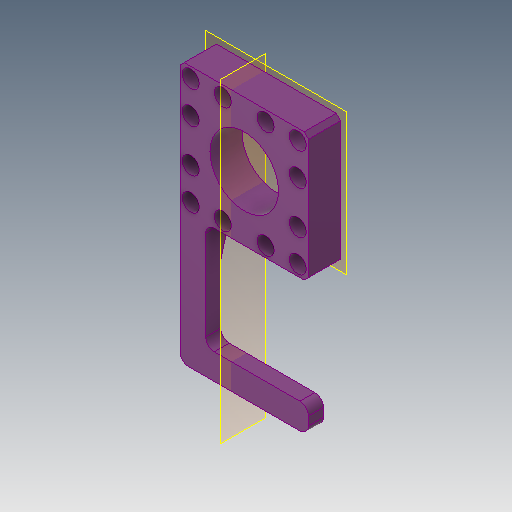
# Autodesk Inventor part: cellSTORM_UC2_Sample_arm
Saved by Autodesk Inventor 2019.4 (Build 234330000, 330)
## iProperties
Created: 2020-12-29
Part Number: cellSTORM_UC2_Sample_arm
Material: Generic
Document SubType Name: Modeling
Designer: diederichbenedict
Density: 1 g/cm^3
Appearance: Smooth - Purple
Author: diederichbenedict
Autodesk Inventor part; units mm, degrees
ref_plane "YZ Plane" through (0, 0, 0) normal (1, 0, 0) x (0, 1, 0)
ref_plane "XZ Plane" through (0, 0, 0) normal (0, 1, 0) x (-1, 0, 0)
ref_plane "XY Plane" through (0, 0, 0) normal (0, 0, 1) x (1, 0, 0)
ref_plane "Work Plane1" through (0, 0, 0) normal (0, 0, 1) x (1, 0, 0)
sketch "Sketch1" plane through (0, 0, 0) normal (0, 0, 1) x (1, 0, 0)
  circle A0 centre (-10, -25) radius 1.45 projected
  circle A1 centre (-10, 25) radius 1.45 projected
  circle A2 centre (10, 25) radius 1.45 projected
  circle A3 centre (10, -25) radius 1.45 projected
  circle A4 centre (-25, 25) radius 2.325 projected
  circle A5 centre (25, -25) radius 2.325 projected
  circle A6 centre (-25, -25) radius 2.325 projected
  circle A7 centre (25, 25) radius 2.325 projected
  line L0 (28, 30) -> (30, 28) projected
  line L1 (28, 30) -> (-28, 30) projected
  line L2 (-30, 28) -> (-28, 30) projected
  line L3 (-30, 28) -> (-30, -28) projected
  line L4 (-28, -30) -> (-30, -28) projected
  line L5 (-28, -30) -> (28, -30) projected
  line L6 (30, -28) -> (28, -30) projected
  line L7 (30, -28) -> (30, 28) projected
  circle A8 centre (-17.5, -17.5) radius 1.95 projected
  circle A9 centre (17.5, 17.5) radius 1.95 projected
  circle A10 centre (17.5, -17.5) radius 1.95 projected
  circle A11 centre (-17.5, 17.5) radius 1.95 projected
  circle A12 centre (0, 0) radius 7.5 projected
  circle A13 centre (-25.33, -75.26) radius 6.15 projected
  circle A14 centre (25, -10) radius 1.45 projected
  circle A15 centre (-25, -10) radius 1.45 projected
  circle A16 centre (-25, 10) radius 1.45 projected
  circle A17 centre (25, 10) radius 1.45 projected
  line L8 (-30, -28) -> (-30, -30)
  line L9 (-30, -30) -> (-28, -30)
  point P0 (0, 0)
  constraints: 4 end point, 1 vertical
extrude "Extrusion1" add sketch "Sketch1" along normal blind 8 contours L0 L7 L6 L5 L4 L3 L2 L1 | L4 L9 L8
sketch "Sketch2" plane through (0, 0, 8) normal (0, 0, 1) x (1, 0, 0)
  circle A0 centre (0, 0) radius 7.5 projected
  circle A1 centre (25, 10) radius 1.45 projected
  circle A2 centre (-25, 10) radius 1.45 projected
  circle A3 centre (-25, -10) radius 1.45 projected
  circle A4 centre (25, -10) radius 1.45 projected
  circle A5 centre (10, -25) radius 1.45 projected
  circle A6 centre (10, 25) radius 1.45 projected
  circle A7 centre (-10, 25) radius 1.45 projected
  circle A8 centre (-10, -25) radius 1.45 projected
  line L0 (-30, -30) -> (28, -30) projected
  line L1 (28, -30) -> (30, -28) projected
  line L2 (30, -28) -> (30, 28) projected
  line L3 (30, 28) -> (28, 30) projected
  line L4 (28, 30) -> (-28, 30) projected
  line L5 (30, -28) -> (30, 28) projected
  line L6 (30, 28) -> (30, -28) projected
  line L7 (-28, 30) -> (-30, 28) projected
  line L8 (-30, 28) -> (-30, -30) projected
  line L9 (-30, -30) -> (-18, -30)
  line L10 (-18, -30) -> (-18, -80)
  line L11 (-18, -80) -> (-30, -80)
  line L12 (-30, -80) -> (-30, -30)
  line L13 (-30, -30) -> (-30, -28)
  line L14 (-30, -28) -> (-28, -30)
  line L15 (-28, -30) -> (-30, -30)
  circle A9 centre (-17.5, 17.5) radius 1.95 projected
  circle A10 centre (-25, 25) radius 2.325 projected
  circle A11 centre (25, 25) radius 2.325 projected
  circle A12 centre (17.5, 17.5) radius 1.95 projected
  circle A13 centre (17.5, -17.5) radius 1.95 projected
  circle A14 centre (25, -25) radius 2.325 projected
  circle A15 centre (-25, -25) radius 2.325 projected
  line L16 (-30, -80) -> (30, -80)
  line L17 (30, -80) -> (30, -92)
  line L18 (30, -92) -> (-30, -92)
  line L19 (-30, -92) -> (-30, -80)
  point P0 (0, 0)
  point P1 (-24.2387, -104)
  dimension "d59" = 12
  dimension "d77" = 12
  constraints: 22 end point, 4 parallel, 2 horizontal, 2 perpendicular, 2 point on line, 1 vertical
  measures "d59" distance of L10.end L11.end
  measures "d77" distance of L16.end L17.end
extrude "Extrusion2" add sketch "Sketch2" along normal blind 7 contours A0 | A1 | A2 | A3 | A4 | A5 | A6 | A7 | A8 | L8 L14 L0 | L0 L10 L11 L12 | L14 L8 L7 L4 L3 L2 L1 L0 | L11 L16 L17 L18 L19 | A9 | A10 | A11 | A12 | A13 | A14 | A15
fillet "Fillet1" radius 4 5 edges at (-18, -30, 11.5) (-30, -92, 11.5) (30, -92, 11.5) (30, -80, 11.5) (-18, -80, 11.5)
sketch "Sketch6" plane through (0, 0, 15) normal (0, 0, 1) x (1, 0, 0)
  line L0 (30, -28) -> (30, 28) projected
  line L1 (30, 28) -> (28, 30) projected
  line L2 (28, 30) -> (-28, 30) projected
  circle A0 centre (-1.1442, -37.6316) radius 2.45
  circle A1 centre (-1.1442, -37.6316) radius 1.45 construction
  line L3 (-14, -30) -> (28, -30) projected
  line L4 (-28, 30) -> (-30, 28) projected
  line L5 (-18, -76) -> (-18, -34) projected
  arc A2 (-14, -30) -> (-18, -34) centre (-14, -34) ccw projected
  line L6 (-26, -92) -> (26, -92) projected
  line L7 (30, -88) -> (30, -84) projected
  line L8 (26, -80) -> (-14, -80) projected
  line L9 (28, -30) -> (30, -28) projected
  arc A3 (30, -84) -> (26, -80) centre (26, -84) ccw projected
  arc A4 (-18, -76) -> (-14, -80) centre (-14, -76) ccw projected
  arc A5 (-30, -88) -> (-26, -92) centre (-26, -88) ccw projected
  arc A6 (26, -92) -> (30, -88) centre (26, -88) ccw projected
  line L10 (-30, 28) -> (-30, -88) projected
  point P0 (0, 0)
  dimension "d27" = 4.9
  constraints: 1 centre point, 1 coincident
  measures "d27" diameter of A0
extrude "Extrusion6" cut sketch "Sketch6" against normal blind 4 contours A0
ref_plane "Work Plane2" through (-6, -91, 19) normal (1, 0, 0) x (0, 0, -1)
sketch "Sketch7" plane through (0, 0, 15) normal (0, 0, 1) x (1, 0, 0)
  circle A0 centre (10, -25) radius 1.45 projected
  circle A1 centre (-10, -25) radius 1.45 projected
  circle A2 centre (-25, -10) radius 1.45 projected
  circle A3 centre (-25, 10) radius 1.45 projected
  circle A4 centre (-10, 25) radius 1.45 projected
  circle A5 centre (10, 25) radius 1.45 projected
  circle A6 centre (25, 10) radius 1.45 projected
  circle A7 centre (25, -10) radius 1.45 projected
  circle A8 centre (-25, 25) radius 2.325 projected
  circle A9 centre (25, 25) radius 2.325 projected
  circle A10 centre (25, -25) radius 2.325 projected
  circle A11 centre (-25, -25) radius 2.325 projected
  point P0 (0, 0)
hole "Hole1" at (-25, -10, 15) at (-25, 10, 15) at (-10, 25, 15) at (10, 25, 15) at (25, 10, 15) at (25, -10, 15) at (10, -25, 15) at (-10, -25, 15) at (-25, 25, 15) at (-25, -25, 15) at (25, -25, 15) at (25, 25, 15) direction (0, 0, -1) diameter 3.2 end through all counterbore diameter 8 counterbore depth 10
sketch "Sketch8" plane through (0, 0, 15) normal (0, 0, 1) x (1, 0, 0)
  circle A0 centre (0, 0) radius 16
  dimension "d41" = 32
  constraints: 1 centre point, 1 coincident
  measures "d41" diameter of A0
extrude "Extrusion7" cut sketch "Sketch8" against normal through all
chamfer "Chamfer3" distance 5 angle 75 1 edges at (-22, -30, 8) measured on face at (14, -30, 7.6667)
body "Solid1"
